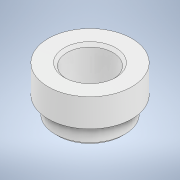
# Autodesk Inventor part: X_end_floating_cup
Saved by Autodesk Inventor 2020 (Build 240168000, 168)
## iProperties
Created: 2022-03-21
Part Number: X_end_floating_cup
Material: Tworzywo sztuczne ABS
Document SubType Name: Modeling
Designer: mikoma
Density: 1.06 g/cm^3
Appearance: Gładki — biały
Mass: 5.39891 g
Surface Area: 32.6298 cm^2
Volume: 5.09331 cm^3
Author: mikoma
Autodesk Inventor part; units mm, degrees
ref_plane "YZ Plane" through (0, 0, 0) normal (1, 0, 0) x (0, 1, 0)
ref_plane "XZ Plane" through (0, 0, 0) normal (0, 1, 0) x (-1, 0, 0)
ref_plane "XY Plane" through (0, 0, 0) normal (0, 0, 1) x (1, 0, 0)
sketch "Szkic1" plane through (0, 0, 0) normal (0, 1, 0) x (-1, 0, 0)
  circle A0 centre (0, 0) radius 15
  circle A1 centre (0, 0) radius 8.25
  circle A2 centre (0, 0) radius 12.5
  dimension "d0" = 30
  dimension "d1" = 16.5
  dimension "d2" = 25
  constraints: 3 centre point, 3 coincident
  measures "d0" diameter of A0
  measures "d1" diameter of A1
  measures "d2" diameter of A2
extrude "Wyciągnięcie proste1" add sketch "Szkic1" along normal blind 17 contours A0 | A1 | A2
extrude "Wyciągnięcie proste2" cut sketch "Szkic1" against normal blind 35 from surface at 17 contours A1
extrude "Wyciągnięcie proste3" cut sketch "Szkic1" along normal blind 7 contours A0
chamfer "Faza1" distance 1 angle 45 2 edges at (12.5, 0, 0) (8.25, 17, 0)
